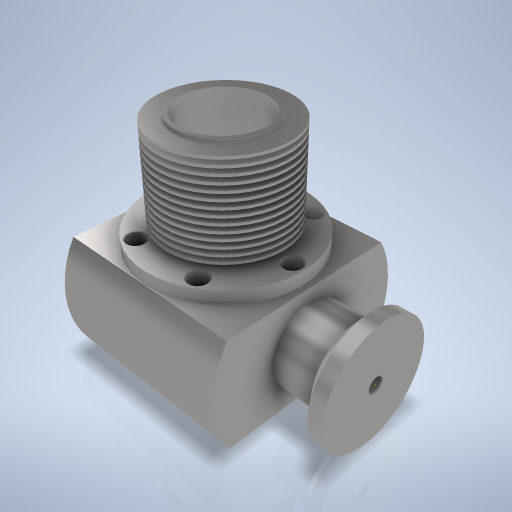
# Autodesk Inventor part: 10
Saved by Autodesk Inventor 2024.2 (Build 282272000, 272)
## iProperties
Created: 2024-05-04
Part Number: 10
Material: Stahl, galvanisiert
Document SubType Name: Modeling
Designer: Fabri
Density: 7.85 g/cm^3
Appearance: Galvanisiert
Author: Fabri
Autodesk Inventor part; units mm, degrees
note: some values were not read from the file. Chosen so that the rebuilt part matches the saved one: direction of "Bohrung5".
ref_plane "YZ Plane" through (0, 0, 0) normal (1, 0, 0) x (0, 1, 0)
ref_plane "XY Plane" through (0, 0, 0) normal (0, 0, 1) x (1, 0, 0)
sketch "Skizze1" plane through (0, 0, 0) normal (0, 1, 0) x (-1, 0, 0)
  line L0 (0, 0) -> (370, 0)
  line L1 (0, 0) -> (0, 88.5)
  line L2 (0, 88.5) -> (20, 88.5)
  line L3 (20, 88.5) -> (40, 60)
  line L4 (40, 60) -> (100, 60)
  line L5 (100, 60) -> (100, 150)
  line L6 (100, 150) -> (370, 150)
  line L7 (370, 150) -> (370, 0)
  point P0 (10, 88.5)
  dimension "d0" = 370
  dimension "d1" = 20
  dimension "d2" = 20
  dimension "d3" = 60
  dimension "d4" = 270
  dimension "d5" = 120
  dimension "d6" = 300
  dimension "d7" = 177
  constraints: 16 end point, 4 perpendicular, 1 horizontal, 1 midpoint, 1 parallel, 1 vertical
  measures "d0" distance of L0.start L0.end
  measures "d1" distance of L1.end L2.end
  measures "d2" horizontal distance of L2.end L3.end
  measures "d3" distance from line of L3.end L5
  measures "d4" distance of L5.end L6.end
  measures "d5" diameter of L4 L0
  measures "d6" diameter of L6 L0
  measures "d7" diameter of point (10, 88.5) L0
revolve "Umdrehung1" add sketch "Skizze1" angle 360 about axis through (0, 0, 0) along (-1, 0, 0)
sketch "Skizze5" plane through (-370, 0, 0) normal (-1, 0, 0) x (0, 0, 1)
  circle A0 centre (0, 0) radius 150 projected
  line L0 (0, 150) -> (0, -150) construction
  line L1 (-80, 126.8858) -> (-80, -126.8858)
  line L2 (80, 126.8858) -> (80, -126.8858)
  dimension "d67" = 80
  dimension "d68" = 80
  constraints: 6 end point, 6 point on circle, 2 vertical, 1 midpoint, 1 parallel
  measures "d67" distance from line of L1 point (0, 0)
  measures "d68" distance from line of L2 point (0, 0)
extrude "Extrusion1" cut sketch "Skizze5" against normal up to surface (270 mm away) contours A0 L2 | L1 A0
sketch "Skizze7" plane through (-370, -126.8858, 80) normal (0, 0, 1) x (1, 0, 0)
  circle A0 centre (135, 126.8858) radius 67.5
  circle A1 centre (135, 126.8858) radius 61.25
  line L0 (270, 0) -> (0, 0) projected
  point P0 (370, 126.8858)
  point P1 (135, 0)
  dimension "d86" = 135
  dimension "d87" = 122.5
  constraints: 2 centre point, 1 coincident, 1 horizontal alignment, 1 midpoint, 1 vertical alignment
  measures "d86" diameter of A0
  measures "d87" diameter of A1
extrude "Extrusion2" add sketch "Skizze7" along normal blind 170
ref_plane "Arbeitsebene1" through (0, 0, 0) normal (0, 1, 0) x (-1, 0, 0)
sketch "Skizze8" plane through (0, 0, 0) normal (0, 1, 0) x (-1, 0, 0)
  line L0 (302.5, 80) -> (302.5, 250) projected
  line L1 (296.25, 250) -> (296.25, 80) projected
  line L2 (302.3881, 80) -> (361.25, 80)
  line L3 (361.25, 80) -> (361.25, 100)
  line L4 (361.25, 100) -> (302.5, 100)
  line L5 (173.75, 250) -> (296.25, 250) projected
  line L6 (296.25, 80) -> (173.75, 80) projected
  line L7 (235, 250) -> (235, -80)
  line L8 (370, -80) -> (100, -80) projected
  line L9 (302.5, 110) -> (328.75, 110)
  line L10 (328.75, 110) -> (328.75, 114)
  line L11 (328.75, 114) -> (302.5, 114)
  line L12 (302.5, 120) -> (328.75, 120)
  line L13 (328.75, 124) -> (302.5, 124)
  line L14 (328.75, 120) -> (328.75, 124)
  line L15 (302.5, 130) -> (328.75, 130)
  line L16 (328.75, 134) -> (302.5, 134)
  line L17 (328.75, 130) -> (328.75, 134)
  line L18 (302.5, 140) -> (328.75, 140)
  line L19 (328.75, 144) -> (302.5, 144)
  line L20 (328.75, 140) -> (328.75, 144)
  line L21 (302.5, 150) -> (328.75, 150)
  line L22 (328.75, 154) -> (302.5, 154)
  line L23 (328.75, 150) -> (328.75, 154)
  line L24 (302.5, 160) -> (328.75, 160)
  line L25 (328.75, 164) -> (302.5, 164)
  line L26 (328.75, 160) -> (328.75, 164)
  line L27 (302.5, 170) -> (328.75, 170)
  line L28 (328.75, 174) -> (302.5, 174)
  line L29 (328.75, 170) -> (328.75, 174)
  line L30 (302.5, 180) -> (328.75, 180)
  line L31 (328.75, 184) -> (302.5, 184)
  line L32 (328.75, 180) -> (328.75, 184)
  line L33 (302.5, 190) -> (328.75, 190)
  line L34 (328.75, 194) -> (302.5, 194)
  line L35 (328.75, 190) -> (328.75, 194)
  line L36 (302.5, 200) -> (328.75, 200)
  line L37 (328.75, 204) -> (302.5, 204)
  line L38 (328.75, 200) -> (328.75, 204)
  line L39 (302.5, 210) -> (328.75, 210)
  line L40 (328.75, 214) -> (302.5, 214)
  line L41 (328.75, 210) -> (328.75, 214)
  line L42 (302.5, 220) -> (328.75, 220)
  line L43 (328.75, 224) -> (302.5, 224)
  line L44 (328.75, 220) -> (328.75, 224)
  line L45 (302.5, 230) -> (328.75, 230)
  line L46 (328.75, 234) -> (302.5, 234)
  line L47 (328.75, 230) -> (328.75, 234)
  line L48 (302.5, 240) -> (328.75, 240)
  line L49 (328.75, 244) -> (302.5, 244)
  line L50 (328.75, 240) -> (328.75, 244)
  line L51 (302.5, 244) -> (302.5, 240)
  line L52 (302.5, 234) -> (302.5, 230)
  line L53 (302.5, 224) -> (302.5, 220)
  line L54 (302.5, 214) -> (302.5, 210)
  line L55 (302.5, 204) -> (302.5, 200)
  line L56 (302.5, 194) -> (302.5, 190)
  line L57 (302.5, 184) -> (302.5, 180)
  line L58 (302.5, 174) -> (302.5, 170)
  line L59 (302.5, 164) -> (302.5, 160)
  line L60 (302.5, 154) -> (302.5, 150)
  line L61 (302.5, 144) -> (302.5, 140)
  line L62 (302.5, 134) -> (302.5, 130)
  line L63 (302.5, 124) -> (302.5, 120)
  line L64 (302.5, 114) -> (302.5, 110)
  line L65 (302.5, 100) -> (302.5, 90)
  line L66 (302.3881, 80) -> (302.3881, 90)
  line L67 (302.3881, 90) -> (302.5, 90)
  point P0 (0, 0)
  point P1 (331.875, 80)
  point P2 (331.875, 100)
  point P3 (328.75, 112)
  point P4 (328.75, 122)
  point P5 (328.75, 132)
  point P6 (328.75, 142)
  point P7 (328.75, 152)
  point P8 (328.75, 162)
  point P9 (328.75, 172)
  point P10 (328.75, 182)
  point P11 (328.75, 192)
  point P12 (328.75, 202)
  point P13 (328.75, 212)
  point P14 (328.75, 222)
  point P15 (328.75, 232)
  point P16 (328.75, 242)
  dimension "d91" = 20
  dimension "d94" = 10
  dimension "d95" = 4
  dimension "d96" = 187.5
  dimension "d97" = 252.5
  dimension "d100" = 10
  constraints: 126 end point, 65 vertical alignment, 26 parallel, 16 vertical, 13 collinear, 5 horizontal, 4 midpoint, 2 perpendicular, 1 point on line, 4 other
  measures "d91" distance of point (331.875, 80) point (331.875, 100)
  measures "d94" distance between parallel lines of L4 L9
  measures "d95" distance between parallel lines of L9 L11
  measures "d96" diameter of point (328.75, 112) L7
  measures "d97" diameter of L3 L7
  measures "d100" distance of L9.start L12.start
revolve "Umdrehung2" add sketch "Skizze8" angle 360 about axis through (-235, 0, 250) along (0, 0, -1) contours L2 L66 L67 L0 | L0 L4 L3 L2 | L0 L11 L10 L9 | L0 L13 L14 L12 | L0 L16 L17 L15 | L0 L19 L20 L18 | L0 L22 L23 L21 | L0 L25 L26 L24 | L0 L28 L29 L27 | L0 L31 L32 L30 | L0 L34 L35 L33 | L0 L37 L38 L36 | L0 L40 L41 L39 | L0 L43 L44 L42 | L0 L46 L47 L45 | L0 L49 L50 L48
sketch "Skizze9" plane through (0, 0, 0) normal (1, 0, 0) x (0, 0, -1)
  circle A0 centre (0, 0) radius 88.5 projected
  constraints: 1 coincident
hole "Bohrung2" at (0, 0, 0) direction (-1, 0, 0) diameter 22.8349 depth 50 thread size "M25x2" class "6H" standard "ISO Metric profile"
sketch "Skizze10" plane through (-370, -126.8858, 80) normal (-1, 0, 0) x (0, 0, 1)
  line L0 (-1.6713, 126.8858) -> (-160, 126.8858) construction
  line L1 (-160, 253.7716) -> (-160, 0) projected
  circle A0 centre (-80, 149.3858) radius 55
  point P0 (-80, 126.8858)
  dimension "d113" = 22.5
  dimension "d114" = 110
  constraints: 2 end point, 1 centre point, 1 coincident, 1 horizontal, 1 midpoint, 1 point on line, 1 vertical alignment
  measures "d113" distance of point (-80, 126.886) A0.centre
  measures "d114" diameter of A0
extrude "Extrusion3" cut sketch "Skizze10" against normal blind 10
sketch "Skizze12" plane through (-360, 22.5, 0) normal (-1, 0, 0) x (0, 0, 1)
  circle A0 centre (0, 0) radius 55 projected
  point P0 (0, -22.5)
  constraints: 1 coincident
hole "Bohrung3" at (-360, 22.5, 0) direction (1, 0, 0) diameter 17.5 depth 115
sketch "Skizze13" plane through (-370, -126.8858, 80) normal (-1, 0, 0) x (0, 0, 1)
  circle A0 centre (-80, 149.3858) radius 8.75 projected
  circle A1 centre (-80, 149.3858) radius 60 construction
  line L0 (-80, 149.3858) -> (-80, 54.9551) construction
  line L1 (-80, 149.3858) -> (-41.7235, 83.0889) construction
  line L2 (-80, 149.3858) -> (-121.2868, 77.875) construction
  point P0 (-80, 126.8858)
  point P1 (-50, 97.4243)
  point P2 (-110, 97.4243)
  dimension "d124" = 120
  dimension "d125" = 30
  dimension "d126" = 30
  constraints: 6 end point, 2 point on circle, 2 point on line, 1 centre point, 1 coincident, 1 vertical
  measures "d124" diameter of A1
  measures "d125" angle of L0 L2
  measures "d126" angle of L0 L1
hole "Bohrung4" at (-370, -29.4615, 30) at (-370, -29.4615, -30) direction (1, 0, 0) diameter 8.376 depth 30 thread size "M10x1.5" class "6H" standard "ISO Metric profile"
pattern_circular "Runde Anordnung2" count 6 over 360 about axis through (-370, 22.5, 0) along (1, 0, 0) of "Bohrung4"
sketch "Skizze15" plane through (0, 0, 0) normal (0, 1, 0) x (-1, 0, 0)
  line L0 (296.25, 80) -> (173.75, 80) projected
  line L1 (108.75, 100) -> (361.25, 100) projected
  line L2 (108.75, 80) -> (361.25, 80) projected
  line L3 (305, 80) -> (305, 90)
  line L4 (108.75, 100) -> (361.25, 100) projected
  line L5 (305, 90) -> (296.25, 90)
  line L6 (296.25, 90) -> (296.25, 80)
  line L7 (305, 80) -> (296.25, 80)
  line L8 (167.5, 240) -> (302.5, 240) projected
  line L9 (235, 240) -> (235, -79.3609)
  point P0 (0, 0)
  dimension "d140" = 10
  dimension "d141" = 140
  constraints: 10 end point, 3 perpendicular, 1 collinear, 1 midpoint, 1 point on line, 1 vertical
  measures "d140" distance of L3.start L3.end
  measures "d141" diameter of L3.start L9
revolve "Umdrehung3" cut sketch "Skizze15" angle 360 about axis through (-235, 0, 240) along (0, 0, -1)
sketch "Skizze16" plane through (0, 0, 0) normal (0, 1, 0) x (-1, 0, 0)
  point P0 (0, 0)
sketch "Skizze6" plane through (-370, -126.8858, 100) normal (0, 0, 1) x (1, 0, 0)
  circle A0 centre (135, 126.8858) radius 107.5 construction
  line L0 (270, 0) -> (0, 0) projected
  line L1 (242.5, 126.8858) -> (27.5, 126.8858) construction
  point P0 (370, 126.8858)
  point P1 (135, 0)
  point P2 (81.25, 33.788)
  point P3 (188.75, 33.788)
  point P4 (242.5, 126.8858)
  point P5 (188.75, 219.9835)
  point P6 (81.25, 219.9835)
  dimension "d71" = 215
  dimension "d84" = 360
  constraints: 2 end point, 2 midpoint, 2 point on circle, 1 centre point, 1 coincident, 1 horizontal, 1 horizontal alignment, 1 vertical alignment, 7 other
  measures "d71" diameter of A0
hole "Bohrung1" at (-342.5, 0, 100) at (-288.75, 93.0977, 100) at (-181.25, 93.0977, 100) at (-127.5, 0, 100) at (-181.25, -93.0977, 100) at (-288.75, -93.0977, 100) direction (0, 0, -1) diameter 30 depth 60
sketch "Skizze17" plane through (-235, 0, 80) normal (0, 0, 1) x (1, 0, 0)
  circle A0 centre (0, 0) radius 61.25 projected
  point P0 (235, 0)
  point P1 (0, 0)
  constraints: 1 coincident
hole "Bohrung5" at (-235, 0, 80) direction (0, 0, -1) diameter 30 depth 160
equation "\"d2\" = d1"
